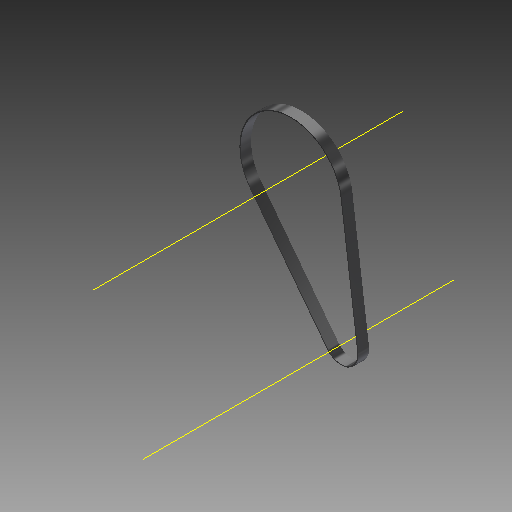
# Autodesk Inventor part: Synchronous Belt
Saved by Autodesk Inventor 2019.4 (Build 234330000, 330)
## iProperties
Created: 2020-03-12
Part Number: Synchronous Belt
Material: Rubber
Document SubType Name: Modeling
Designer: Mark
Density: 0.93 g/cm^3
Appearance: Rubber - Black - Version 1.1
Mass: 4.23149 g
Surface Area: 100.1 cm^2
Volume: 4.54999 cm^3
CustomPartVersion: 1
Author: Mark
Autodesk Inventor part; units mm, degrees
sketch "Sketch Path" plane through (0, 0, 0) normal (0, 0, 1) x (1, 0, 0)
  arc A0 (34.6002, -74.1806) -> (63.0103, -62.4065) centre (47.2331, -64.5) ccw
  arc A1 (47.3316, 55.7507) -> (-37.8986, 20.4284) centre (0, 49.4701) ccw
  line L0 (47.3316, 55.7507) -> (63.0103, -62.4065)
  line L1 (34.6002, -74.1806) -> (-37.8986, 20.4284)
  constraints: 4 end point, 4 point on circle, 2 centre point
ref_plane "Cross Section Plane" through (63.0103, -62.4065, 0) normal (-0.1315, 0.9913, 0) x (0, 0, 1)
ref_plane "Work Plane2" through (47.2331, -64.5, 0) normal (-1, 0, 0) x (0, 0, 1)
ref_plane "Work Plane3" through (0, 49.4701, 0) normal (0.5879, -0.8089, 0) x (0, 0, 1)
sketch "Cross Section" plane through (63.0103, -62.4065, 0) normal (-0.1315, 0.9913, 0) x (0, 0, 1)
  line L0 (-5, 0.5) -> (5, 0.5)
  line L1 (5, 0.5) -> (5, -0.5)
  line L2 (5, -0.5) -> (-5, -0.5)
  line L3 (-5, -0.5) -> (-5, 0.5)
  line L4 (-5, 0) -> (5, 0) construction
  point P0 (0, 0)
  point P1 (0, 0)
  dimension "d0" = 10
  dimension "d4" = 0.5
  dimension "d5" = 0.5
  constraints: 10 end point, 3 midpoint, 2 parallel, 1 coincident, 1 horizontal, 1 perpendicular, 1 other
  measures "d0" distance between parallel lines of L1 L3
  measures "d4" distance between parallel lines of L2 L4
  measures "d5" distance between parallel lines of L4 L0
sweep "Belt" add profiles "Cross Section" path "Sketch Path"
equation "\"d0\" = da_B"
equation "\"d4\" = da_a"
equation "\"d5\" = da_a2"
equation "\"da_B\" = 10"
equation "\"da_pb\" = 5"
equation "\"da_L\" = 454.99929"
equation "\"da_a\" = 0.5"
equation "\"da_S\" = 2.65"
equation "\"da_Beta\" = 20deg"
equation "\"da_Ht\" = 1.2"
equation "\"da_H\" = 2.2"
equation "\"da_a2\" = 0.5"
body "Solid1"
